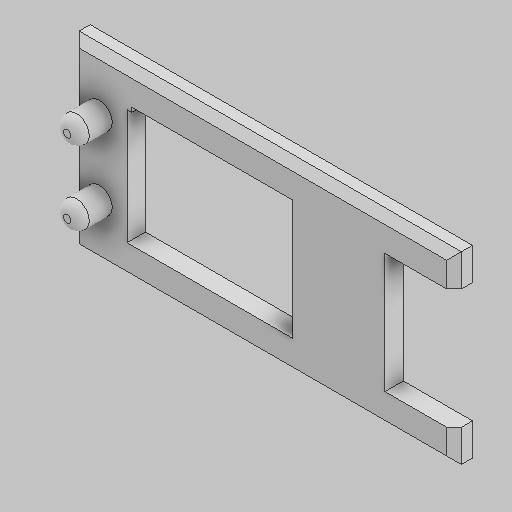
# Autodesk Inventor part: Modules_cover
Saved by Autodesk Inventor 2026.1 (Build 301233020, 233B)
## iProperties
Created: 2026-01-23
Part Number: Modules_cover
Material: Generic
Document SubType Name: Modeling
Designer: samuel
Density: 1 g/cm^3
Appearance: Default
Author: samuel
Autodesk Inventor part; units mm, degrees
ref_plane "YZ Plane" through (0, 0, 0) normal (1, 0, 0) x (0, 1, 0)
ref_plane "XZ Plane" through (0, 0, 0) normal (0, 1, 0) x (-1, 0, 0)
ref_plane "XY Plane" through (0, 0, 0) normal (0, 0, 1) x (1, 0, 0)
sketch "Sketch1" plane through (0, 0, 0) normal (0, 0, 1) x (1, 0, 0)
  line L0 (-20.75, -10) -> (20.75, -10)
  line L1 (20.75, -10) -> (20.75, 10)
  line L2 (20.75, 10) -> (-20.75, 10)
  line L3 (-20.75, 10) -> (-20.75, -10)
  line L4 (-20.75, -10) -> (20.75, 10) construction
  line L5 (20.75, -10) -> (-20.75, 10) construction
  circle A0 centre (-17.75, 4) radius 1.4
  circle A1 centre (-17.75, -4) radius 1.4
  point P0 (0, 0)
  dimension "d0" = 41.5
  dimension "d1" = 20
  dimension "d2" = 2.8
  dimension "d3" = 2.8
  dimension "d4" = 6
  dimension "d5" = 6
  dimension "d6" = 3
  dimension "d7" = 3
  constraints: 12 end point, 2 centre point, 2 midpoint, 2 parallel, 1 horizontal, 1 perpendicular
  measures "d0" distance of L2.end L1.end
  measures "d1" distance of L1.end L0.end
  measures "d2" diameter of A0
  measures "d3" diameter of A1
  measures "d4" distance from line of L2 A0.centre
  measures "d5" distance from line of L0 A1.centre
  measures "d6" distance from line of L3 A1.centre
  measures "d7" distance from line of L3 A0.centre
extrude "Extrusion1" add sketch "Sketch1" along normal blind 2
extrude "Extrusion2" add sketch "Sketch1" along normal blind 5.5 contours A0 | A1
fillet "Fillet1" radius 1 2 edges at (-19.15, -4, 5.5) (-19.15, 4, 5.5)
chamfer "Chamfer1" distance 0.8 angle 45 4 edges at (-20.75, 0, 2) (0, 10, 2) (0, -10, 2) (20.75, 0, 2)
sketch "Sketch2" plane through (0, 0, 2) normal (0, 0, 1) x (1, 0, 0)
  line L0 (20.75, -10) -> (20.75, 10) projected
  line L1 (20.75, -6.5) -> (-14.25, -6.5)
  line L2 (-14.25, -6.5) -> (-14.25, 6.5)
  line L3 (-14.25, 6.5) -> (20.75, 6.5)
  line L4 (20.75, 6.5) -> (20.75, -6.5)
  line L5 (20.75, 10) -> (-20.75, 10) projected
  line L6 (-20.75, -10) -> (20.75, -10) projected
  line L7 (-20.75, 10) -> (-20.75, -10) projected
  line L8 (20.75, 6.5) -> (13.25, 6.5)
  line L9 (13.25, 6.5) -> (13.25, -6.5)
  line L10 (13.25, -6.5) -> (20.75, -6.5)
  line L11 (20.75, -6.5) -> (20.75, 6.5)
  line L12 (13.25, -6.5) -> (3.25, -6.5)
  line L13 (3.25, -6.5) -> (3.25, 6.5)
  line L14 (3.25, 6.5) -> (13.25, 6.5)
  line L15 (13.25, 6.5) -> (13.25, -6.5)
  line L16 (-14.25, -6.5) -> (-14.75, -6.5)
  line L17 (-14.75, -6.5) -> (-14.75, 6)
  line L18 (-14.75, 6) -> (-14.25, 6)
  line L19 (-14.25, 6) -> (-14.25, -6.5)
  point P0 (0, 0)
  point P1 (20.75, 6.5)
  point P2 (3.25, -6.5)
  point P3 (-14.5, 6)
  point P4 (-14.5, 6)
  dimension "d16" = 3.5
  dimension "d17" = 3.5
  dimension "d18" = 6.5
  dimension "d19" = 7.5
  dimension "d20" = 10
  dimension "d23" = 0.5
  constraints: 32 end point, 8 parallel, 4 horizontal, 4 perpendicular, 2 point on line, 1 midpoint
  measures "d16" distance between parallel lines of L5 L3
  measures "d17" distance between parallel lines of L6 L1
  measures "d18" distance between parallel lines of L7 L2
  measures "d19" distance of L10.end L9.end
  measures "d20" distance of L13.end L14.end
  measures "d23" distance of L17.end L18.end
extrude "Extrusion3" cut sketch "Sketch2" against normal blind 2.5 contours L1 L9 L3 L0 | L1 L2 L3 L13 | L16 L17 L18 L2
body "Solid1"
